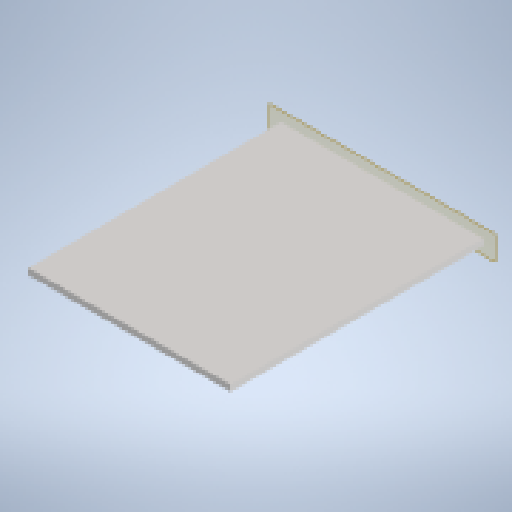
# Autodesk Inventor part: Опорная грань
Saved by Autodesk Inventor 2023.1 (Build 271208000, 208)
## iProperties
Created: 2024-11-20
Part Number: Опорная грань
Material: Типовые
Document SubType Name: Modeling
Designer: DELL
Density: 1 g/cm^3
Appearance: По умолчанию
Author: DELL
Autodesk Inventor part; units mm, degrees
ref_plane "YZ Plane" through (0, 0, 0) normal (1, 0, 0) x (0, 1, 0)
ref_plane "XZ Plane" through (0, 0, 0) normal (0, 1, 0) x (-1, 0, 0)
ref_plane "XY Plane" through (0, 0, 0) normal (0, 0, 1) x (1, 0, 0)
ref_plane "РабПлоскость1" through (72.1794, 3.1188, -6) normal (0, 0, 1) x (1, 0, 0)
sketch "Эскиз1" plane through (72.1794, 3.1188, -6) normal (0, 0, 1) x (1, 0, 0)
  ellipse E0 centre (-72.1794, -3.1188) end of major axis (-192.177, -2.3565) minor radius 79.9991 projected
  line L0 (27.8206, -1.1188) -> (-172.1794, -1.1188)
  line L1 (-172.1794, -1.1188) -> (-172.1794, -5.1188)
  line L2 (-172.1794, -5.1188) -> (27.8206, -5.1188)
  line L3 (27.8206, -5.1188) -> (27.8206, -1.1188)
  line L4 (27.8206, -1.1188) -> (-172.1794, -5.1188) construction
  line L5 (-172.1794, -1.1188) -> (27.8206, -5.1188) construction
  line L6 (-246.043, 0) -> (103.957, 0) projected
  dimension "d4" = 200
  dimension "d5" = 4
  constraints: 12 end point, 2 midpoint, 2 parallel, 1 horizontal, 1 perpendicular, 1 other
  measures "d4" distance of L2.end L1.end
  measures "d5" distance of L1.end L0.end
extrude "Выдавливание1" add sketch "Эскиз1" along normal blind 250 contours L3 L2 L1 L0
